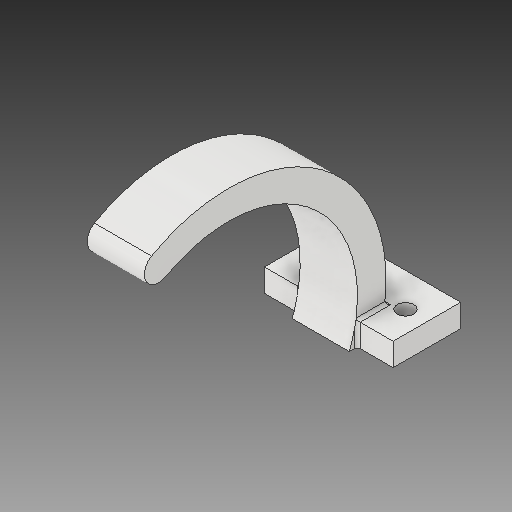
# Autodesk Inventor part: TopBracket
Saved by Autodesk Inventor 2018 (Build 220112000, 112)
## iProperties
Created: 2019-04-15
Part Number: TopBracket
Material: Generic
Document SubType Name: Modeling
Designer: anirudh
Density: 1 g/cm^3
Appearance: White
Mass: 8.06105 g
Surface Area: 41.8583 cm^2
Volume: 8.06105 cm^3
Author: anirudh
Autodesk Inventor part; units mm, degrees
ref_plane "YZ Plane" through (0, 0, 0) normal (1, 0, 0) x (0, 1, 0)
ref_plane "XZ Plane" through (0, 0, 0) normal (0, 1, 0) x (-1, 0, 0)
ref_plane "XY Plane" through (0, 0, 0) normal (0, 0, 1) x (1, 0, 0)
sketch "Sketch1" plane through (0, 0, 0) normal (1, 0, 0) x (0, 1, 0)
  arc A0 (-9.892, -26.808188) -> (23.379545, 16.42947) centre (0, 0) ccw
  line L0 (-9.892, -26.808188) -> (-9.892, -43.575)
  line L1 (-9.892, -43.575) -> (-4.812, -43.575)
  line L2 (-4.812, -43.575) -> (-4.812, -34.591911)
  line L3 (-4.812, -43.575) -> (-4.812, -34.591911)
  line L4 (28.575, 20.080463) -> (23.379545, 16.42947)
  arc A1 (-4.812, -34.591911) -> (28.575, 20.080463) centre (0, 0) ccw
  dimension "d0" = 57.15
  constraints: 10 end point, 4 point on circle, 2 centre point, 1 coincident, 1 perpendicular
  measures "d0" diameter of A0
extrude "Extrusion1" add sketch "Sketch1" along normal blind 9.525
sketch "Sketch2" plane through (0, -4.812, -34.591911) normal (0, 1, 0) x (1, 0, 0)
  line L0 (0, -7.783722) -> (0, 8.983089)
  line L1 (0, 8.983089) -> (-9.525, 8.983089)
  line L2 (-9.525, 8.983089) -> (-9.525, -6.016911)
  line L3 (-9.525, -6.016911) -> (0, -6.016911)
  line L4 (0, -6.016911) -> (0, 8.983089)
  line L5 (0, 8.983089) -> (9.525, 8.983089)
  line L6 (9.525, 8.983089) -> (19.05, 8.983089)
  line L7 (19.05, 8.983089) -> (19.05, -6.016911)
  line L8 (19.05, -6.016911) -> (9.525, -6.016911)
  line L9 (9.525, -6.016911) -> (9.525, 8.983089)
  line L10 (9.525, -7.783722) -> (9.525, 8.983089)
  circle A0 centre (-4.7625, 1.483089) radius 1.85
  circle A1 centre (14.2875, 1.483089) radius 1.85
  point P0 (0, -34.591911)
  dimension "d11" = 9.525
  dimension "d12" = 15
  dimension "d13" = 9.525
  dimension "d14" = 3.7
  dimension "d15" = 3.7
  constraints: 16 end point, 4 parallel, 2 centre point, 2 horizontal, 2 perpendicular, 1 point on line
  measures "d11" distance of L3.end L2.end
  measures "d12" distance of L2.end L1.end
  measures "d13" distance of L7.end L8.end
  measures "d14" diameter of A0
  measures "d15" diameter of A1
extrude "Extrusion2" add sketch "Sketch2" against normal blind 5.08
ref_plane "Work Plane1" through (4.7625, 0, 0) normal (1, 0, 0) x (0, 0, -1)
sketch "Sketch3" plane through (4.7625, 0, 0) normal (1, 0, 0) x (0, 0, -1)
  line L0 (-20.080463, 28.575) -> (-16.42947, 23.379545)
  arc A0 (26.808188, -9.892) -> (-16.42947, 23.379545) centre (0, 0) ccw
  arc A1 (33.494835, -9.892) -> (-20.080463, 28.575) centre (0, 0) ccw
  arc A2 (34.591911, -4.812) -> (-20.080463, 28.575) centre (0, 0) ccw
  line L1 (-20.080463, 28.575) -> (-16.42947, 23.379545)
  line L2 (26.808188, -9.892) -> (28.575, -9.892)
  line L3 (26.808188, -9.892) -> (33.494835, -9.892)
  constraints: 4 end point, 4 point on circle, 2 centre point, 2 coincident, 2 collinear
extrude "Extrusion3" add sketch "Sketch3" along normal mid plane 12.7
fillet "Fillet4" radius 3.175 2 edges at (4.7625, 28.575, 20.0805) (4.7625, 23.3795, 16.4295)
fillet "Fillet5" radius 0.635 5 edges at (11.1125, -7.352, -28.575) (-1.5875, -7.352, -28.575) (-1.5875, -4.812, -31.5835) (4.7625, -4.812, -34.5919) (11.1125, -4.812, -31.5835)
body "Solid1"
